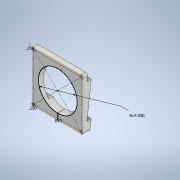
# Autodesk Inventor part: ventForDryer02
Saved by Autodesk Inventor 2022.1 (Build 261234020, 234B)
## iProperties
Created: 2020-08-29
Part Number: ventForDryer02
Material: Generic
Document SubType Name: Modeling
Designer: robst
Density: 1 g/cm^3
Appearance: Default
Author: robst
Autodesk Inventor part; units mm, degrees
ref_plane "YZ Plane" through (0, 0, 0) normal (1, 0, 0) x (0, 1, 0)
ref_plane "XZ Plane" through (0, 0, 0) normal (0, 1, 0) x (-1, 0, 0)
ref_plane "XY Plane" through (0, 0, 0) normal (0, 0, 1) x (1, 0, 0)
sketch "Sketch4" plane through (0, 0, 0) normal (1, 0, 0) x (0, 1, 0)
  line L0 (0, 0) -> (0, -12.7)
  line L1 (0, -12.7) -> (-101.6, 0)
  line L2 (-101.6, 0) -> (-101.6, -12.7)
  line L3 (-101.6, -12.7) -> (-203.2, 0)
  line L4 (-203.2, 0) -> (-203.2, -12.7)
  line L5 (-203.2, -12.7) -> (-304.8, 0)
  line L6 (-82.55, -2.3812) -> (-82.55, 10.3187)
  line L7 (-82.55, 10.3187) -> (-234.95, 10.3187)
  line L8 (-234.95, 10.3187) -> (-234.95, -8.7313)
  dimension "d28" = 12.7
  dimension "d29" = 101.6
  dimension "d30" = 101.6
  dimension "d31" = 12.7
  dimension "d32" = 101.6
  dimension "d33" = 152.4
  dimension "d34" = 12.7
  dimension "d35" = 19.05
  constraints: 18 end point, 5 vertical, 2 point on line, 1 perpendicular
  measures "d28" distance of L0.start L0.end
  measures "d29" distance of L1.end L0.start
  measures "d30" distance of L3.end L1.end
  measures "d31" distance of L3.end L4.end
  measures "d32" distance of L5.end L3.end
  measures "d33" distance of L6.end L7.end
  measures "d34" distance of L6.start L6.end
  measures "d35" distance from line of L1.end L6
extrude "Extrusion3" add sketch "Sketch4" along normal mid plane 152.4
sketch "Sketch5" plane through (-76.2, -234.95, 10.3187) normal (0, 0, 1) x (1, 0, 0)
  line L0 (0, 0) -> (0, 152.4) construction
  line L1 (0, 152.4) -> (152.3647, 0) construction
  line L2 (152.4, 152.4) -> (152.4, 0) construction
  line L3 (0, 0) -> (152.4, 0) construction
  line L4 (152.4, 152.4) -> (0, 0) construction
  line L5 (6.35, 6.35) -> (146.05, 6.35) construction
  line L6 (146.05, 6.35) -> (146.05, 146.05) construction
  line L7 (146.05, 146.05) -> (6.35, 146.05) construction
  line L8 (6.35, 146.05) -> (6.35, 6.35) construction
  line L9 (6.35, 6.35) -> (146.05, 146.05) construction
  line L10 (146.05, 6.35) -> (6.35, 146.05) construction
  line L11 (0, 152.4) -> (152.4, 152.4) construction
  circle A0 centre (76.2, 76.2) radius 57.15
  line L12 (76.2, 19.05) -> (76.2, 0) construction
  line L13 (0, 0) -> (152.4, 0) construction
  line L14 (76.454, 0) -> (76.454, 19.0506)
  line L15 (75.946, 0) -> (75.946, 19.0506)
  line L16 (75.946, 0) -> (76.454, 0)
  point P0 (76.2, 234.95)
  point P1 (75.946, 19.0506)
  dimension "d38" = 6.35
  dimension "d39" = 6.35
  dimension "d40" = 114.3
  dimension "d51" = 0.254
  constraints: 24 end point, 5 coincident, 4 midpoint, 2 parallel, 2 perpendicular, 2 point on circle, 2 symmetric about line, 1 centre point, 1 collinear, 1 horizontal, 1 point on line
  measures "d38" distance between parallel lines of L7 L11
  measures "d39" distance between parallel lines of L0 L8
  measures "d40" diameter of A0
  measures "d51" distance between parallel lines of L14 L12
extrude "Extrusion4" cut sketch "Sketch5" against normal through all contours A0
hole "Hole2" at (-69.85, -88.9, 10.3187) at (69.85, -88.9, 10.3187) at (69.85, -228.6, 10.3187) at (-69.85, -228.6, 10.3187) direction (0, 0, -1) diameter 6.7564 end through all clearance for "Hex Machine Screw" size "1/4" standard "Ansi Unified Screw Threads"
fillet "Fillet2" radius 6.35 4 edges at (76.2, -82.55, 3.9687) (-76.2, -82.55, 3.9687) (76.2, -234.95, 0.7937) (-76.2, -234.95, 0.7937)
extrude "Extrusion5" cut sketch "Sketch5" against normal through all contours A0 L14 L16 L15
equation "\"d36\" = outsideWidthOfVent"
equation "\"d40\" = ventHole"
equation "\"d50\" = ventRadius"
equation "\"sidingHeight\" = 101.6"
equation "\"sidingDepth\" = 12.7"
equation "\"radiusOfCurvature\" = 609.6"
equation "\"outsideWidthOfVent\" = 152.4"
equation "\"wallThicknessOfVent\" = 19.05"
equation "\"holeOffset\" = 6.35"
equation "\"ventHole\" = 114.3"
equation "\"ventRadius\" = 6.35"
body "Solid1"
body "Solid2"
